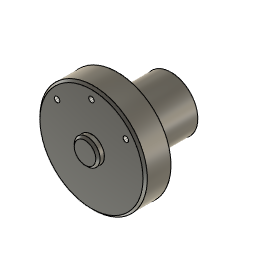
Housing Fixture v1 (Autodesk Fusion 360 design; units mm, degrees)
Autodesk Fusion 360 part; units mm, degrees
sketch "Sketch1" plane through (0, 0, 0) normal (0, 1, 0) x (1, 0, 0)
  circle A0 centre (0, 0) radius 6
  circle A1 centre (0, 0) radius 25
  circle A2 centre (0, 0) radius 12.5
  circle A3 centre (0, 0) radius 20 construction
  circle A4 centre (16, -12) radius 1.5
  line L0 (0, -25) -> (0, 0) construction
  circle A5 centre (-16, -12) radius 1.5
  circle A6 centre (0, -20) radius 1.5
  dimension "d10" = 12
  dimension "d11" = 50
  dimension "d12" = 25
  dimension "d13" = 40
  dimension "d14" = 3
  dimension "d16" = 12
  dimension "d17" = 3
  constraint coincident A0.centre A1.centre
  constraint concentric A1 A2
  constraint coincident A3 A4.centre
  constraint coincident A1 L0.start
  constraint vertical L0
  constraint symmetric A4 L0 A5
  constraint coincident A3 A6.centre
  constraint coincident L0 A6.centre
  measures "d10" diameter of A0
  measures "d11" diameter of A1
  measures "d12" diameter of A2
  measures "d13" diameter of A3
  measures "d14" diameter of A4
  measures "d16" vertical distance of A0.centre A4.centre
  measures "d17" diameter of A6
extrude "Extrude1" add sketch "Sketch1" against normal blind 3 contours A0 makes body 1
extrude "Extrude2" add sketch "Sketch1" along normal blind 37 separate body contours A2 makes body 2
extrude "Extrude3" add sketch "Sketch1" along normal blind 12 contours A1 bodies 2
chamfer "Chamfer1" distance 1 angle 45 2 edges at (-5.594, -3, -2.1697) (-23.3082, 0, 9.0404) on bodies 1 2
thread "Thread1" "ISO Metric profile 3.0 M3x0.5 6H" major diameter 3.086 minor diameter 2.529 pitch 0.5 angle 60 resizes the face on face at (-14.5019, 8, 12.0748) on bodies 2
thread "Thread2" "ISO Metric profile 3.0 M3x0.5 6H" major diameter 3.086 minor diameter 2.529 pitch 0.5 angle 60 resizes the face on face at (1.4981, 4, 19.9252) on face at (17.4981, 4, 11.9252) on face at (-14.7371, 4, 11.937) on bodies 2
equation "knob_height = 3 mm"
equation "chamfer = 1 mm"
equation "base_height = 12 mm"
equation "center_height = 25 mm"
equation "center_diameter = 25 mm"
equation "knob_diameter = 12 mm"
equation "threaded_hole_distance_from_center = 40 mm"
equation "base_diameter = 50 mm"
equation "threaded_hole_diameter = 3 mm"
equation "d10 = knob_diameter"
equation "d11 = base_diameter"
equation "d12 = center_diameter"
equation "d13 = threaded_hole_distance_from_center"
equation "d14 = threaded_hole_diameter"
equation "threaded_hole_height = 12 mm"
equation "d16 = threaded_hole_height"
equation "d17 = threaded_hole_diameter"
equation "d18 = -knob_height"
equation "d20 = center_height + base_height"
equation "d22 = base_height"
equation "d24 = chamfer"
